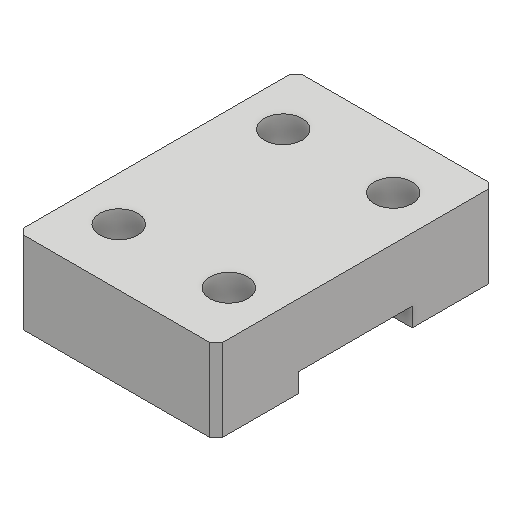
# Autodesk Inventor part: 3DP_ABS_X_Axis_Timing_Belt_Clamp
Saved by Autodesk Inventor 2026.1 (Build 301233000, 233)
## iProperties
Created: 2016-06-18
Part Number: 3DP_ABS_X_Axis_Timing_Belt_Clamp
Material: Ogólny
Document SubType Name: Modeling
Designer: Andrzej
Density: 1 g/cm^3
Appearance: Domyślna
Mass: 1.88495 g
Surface Area: 14.8746 cm^2
Volume: 1.88495 cm^3
Author: Andrzej
Autodesk Inventor part; units mm, degrees
ref_plane "YZ Plane" through (0, 0, 0) normal (1, 0, 0) x (0, 1, 0)
ref_plane "XZ Plane" through (0, 0, 0) normal (0, 1, 0) x (-1, 0, 0)
ref_plane "XY Plane" through (0, 0, 0) normal (0, 0, 1) x (1, 0, 0)
sketch "Szkic1" plane through (0, 0, 0) normal (0, 0, 1) x (1, 0, 0)
  line L0 (-11.2555, 18.1319) -> (4.4445, 18.1319)
  line L1 (4.4445, 18.1319) -> (4.4445, -3.8681)
  line L2 (4.4445, -3.8681) -> (-11.2555, -3.8681)
  line L3 (-11.2555, -3.8681) -> (-11.2555, 18.1319)
  line L4 (-11.2555, 2.6319) -> (4.4445, 2.6319)
  line L5 (-11.2555, 11.6319) -> (4.4445, 11.6319)
  point P0 (0, 0)
  dimension "d0" = 15.7
  dimension "d1" = 22
  dimension "d2" = 9
  dimension "d3" = 6.5
  dimension "d4" = 6.5
  constraints: 12 end point, 4 point on line, 3 perpendicular, 2 parallel, 1 horizontal
  measures "d0" distance of L1.end L2.end
  measures "d1" distance of L2.end L0.start
  measures "d2" distance between parallel lines of L5 L4
  measures "d3" distance between parallel lines of L0 L5
  measures "d4" distance between parallel lines of L2 L4
extrude "Wyciągnięcie proste1" add sketch "Szkic1" along normal blind 1.5 contours L0 L1 L5 L3 | L4 L1 L2 L3
sketch "Szkic2" plane through (0, 0, 1.5) normal (0, 0, 1) x (1, 0, 0)
  line L0 (-11.2555, 18.1319) -> (-11.2555, 11.6319) projected
  line L1 (-11.2555, 18.1319) -> (-11.2555, 11.6319) projected
  line L2 (-11.2555, 11.6319) -> (4.4445, 11.6319) projected
  line L3 (4.4445, 11.6319) -> (4.4445, 18.1319) projected
  line L4 (4.4445, 18.1319) -> (-11.2555, 18.1319) projected
  line L5 (4.4445, -3.8681) -> (4.4445, 2.6319) projected
  line L6 (4.4445, 2.6319) -> (-11.2555, 2.6319) projected
  line L7 (-11.2555, 2.6319) -> (-11.2555, -3.8681) projected
  line L8 (-11.2555, -3.8681) -> (4.4445, -3.8681) projected
  line L9 (4.4445, 18.1319) -> (-11.2555, 18.1319) projected
  line L10 (-11.2555, 18.1319) -> (4.4445, 18.1319)
  line L11 (4.4445, 18.1319) -> (4.4445, -3.8681)
  line L12 (4.4445, -3.8681) -> (-11.2555, -3.8681)
  line L13 (-11.2555, -3.8681) -> (-11.2555, 18.1319)
  point P0 (0, 0)
  constraints: 8 end point, 2 parallel, 1 horizontal, 1 perpendicular
extrude "Wyciągnięcie proste2" add sketch "Szkic2" along normal blind 5
sketch "Szkic3" plane through (0, 0, 6.5) normal (0, 0, 1) x (1, 0, 0)
  line L0 (-11.2555, 11.6319) -> (4.4445, 11.6319) projected
  line L1 (4.4445, 2.6319) -> (-11.2555, 2.6319) projected
  line L2 (-11.2555, 18.1319) -> (-11.2555, -3.8681) projected
  line L3 (-11.2555, -3.8681) -> (4.4445, -3.8681) projected
  line L4 (4.4445, -3.8681) -> (4.4445, 18.1319) projected
  line L5 (4.4445, 18.1319) -> (-11.2555, 18.1319) projected
  point P0 (0, 0)
  point P1 (-7.7555, 13.6319)
  point P2 (0.9445, 13.6319)
  point P3 (-7.7555, 0.6319)
  point P4 (0.9445, 0.6319)
  dimension "d9" = 2
  dimension "d10" = 2
  dimension "d11" = 2
  dimension "d12" = 2
  dimension "d13" = 15.7
  dimension "d14" = 3.5
  dimension "d15" = 3.5
  dimension "d16" = 3.5
  dimension "d17" = 3.5
  measures "d9" distance from line of L0 point (-7.756, 13.632)
  measures "d10" distance from line of L0 point (0.944, 13.632)
  measures "d11" distance from line of L1 point (0.944, 0.632)
  measures "d12" distance from line of L1 point (-7.756, 0.632)
  measures "d13" distance of L4.end L2.start
  measures "d14" distance from line of point (-7.756, 13.632) L2
  measures "d15" distance from line of L4 point (0.944, 13.632)
  measures "d16" distance from line of L4 point (0.944, 0.632)
  measures "d17" distance from line of L2 point (-7.756, 0.632)
hole "Otwór1" at (-7.7555, 13.6319, 6.5) at (0.9445, 13.6319, 6.5) at (-7.7555, 0.6319, 6.5) at (0.9445, 0.6319, 6.5) direction (0, 0, -1) diameter 3 end through all
sketch "Szkic5" plane through (-11.2555, 2.6319, 0) normal (0, 1, 0) x (1, 0, 0)
  line L0 (0, 0) -> (15.7, 0) projected
  line L1 (15.7, 0) -> (15.7, -6.5) projected
  line L2 (0, -6.5) -> (15.7, -6.5) projected
  line L3 (0, 0) -> (0, -6.5) projected
  line L4 (12.8, -0.5) -> (12, -0.5)
  line L5 (12, -0.5) -> (12, -1.5)
  line L6 (10.8, -0.5) -> (10.8, -1.5)
  line L7 (10.8, -0.5) -> (10, -0.5)
  line L8 (10, -0.5) -> (10, -1.5)
  line L9 (8.8, -0.5) -> (8.8, -1.5)
  line L10 (8.8, -0.5) -> (8, -0.5)
  line L11 (8, -0.5) -> (8, -1.5)
  line L12 (6.8, -0.5) -> (6.8, -1.5)
  line L13 (6.8, -0.5) -> (6, -0.5)
  line L14 (6, -0.5) -> (6, -1.5)
  line L15 (4.8, -0.5) -> (4.8, -1.5)
  line L16 (4.8, -0.5) -> (4, -0.5)
  line L17 (4, -0.5) -> (4, -1.5)
  line L18 (2.8, -0.5) -> (2.8, -1.5)
  line L19 (2.8, -0.5) -> (2, -0.5)
  line L20 (2, -0.5) -> (2, -1.5)
  line L21 (0.8, -0.5) -> (0.8, -1.5)
  line L22 (0.8, -0.5) -> (0, -0.5)
  line L23 (12.8, -0.5) -> (12.8, -1.5)
  line L24 (14, -1.5) -> (14, -0.5)
  line L25 (14, -0.5) -> (14.8, -0.5)
  line L26 (14.8, -0.5) -> (14.8, -1.5)
  line L27 (0, -1.5) -> (0.8, -1.5)
  line L28 (2, -1.5) -> (2.8, -1.5)
  line L29 (4, -1.5) -> (4.8, -1.5)
  line L30 (6, -1.5) -> (6.8, -1.5)
  line L31 (8, -1.5) -> (8.8, -1.5)
  line L32 (10, -1.5) -> (10.8, -1.5)
  line L33 (12, -1.5) -> (12.8, -1.5)
  line L34 (14, -1.5) -> (14.8, -1.5)
  line L35 (0, -1.5) -> (0, -0.5)
  line L36 (0, 0) -> (0, -6.5) projected
  point P0 (11.2555, 0)
  dimension "d27" = 0.8
  dimension "d28" = 1.2
  dimension "d41" = 1
  dimension "d42" = 0.5
  dimension "d43" = 0.5
  dimension "d44" = 0.5
  dimension "d45" = 0.5
  dimension "d46" = 0.5
  dimension "d47" = 0.5
  dimension "d48" = 0.5
  dimension "d49" = 0.5
  dimension "d50" = 1
  constraints: 64 end point, 16 perpendicular, 9 horizontal, 1 collinear, 1 point on line, 1 vertical
  measures "d27" distance of L24.end L25.end
  measures "d28" distance between parallel lines of L24 L23
  measures "d41" distance of L25.end L26.end
  measures "d42" distance between parallel lines of L0 L25
  measures "d43" distance between parallel lines of L0 L4
  measures "d44" distance between parallel lines of L0 L7
  measures "d45" distance between parallel lines of L0 L10
  measures "d46" distance between parallel lines of L0 L13
  measures "d47" distance between parallel lines of L0 L16
  measures "d48" distance between parallel lines of L0 L19
  measures "d49" distance between parallel lines of L0 L22
  measures "d50" distance between parallel lines of L22 L27
extrude "Wyciągnięcie proste3" add sketch "Szkic5" along normal blind 9 contours L22 L21 L27 L3 | L23 L33 L5 L4 | L6 L32 L8 L7 | L9 L31 L11 L10 | L12 L30 L14 L13 | L15 L29 L17 L16 | L18 L28 L20 L19 | L24 L25 L26 L34
fillet "Zaokrąglenie1" radius 0.2 16 edges at (-9.2555, 7.1319, 0.5) (-8.4555, 7.1319, 0.5) (-7.2555, 7.1319, 0.5) (-6.4555, 7.1319, 0.5) (-5.2555, 7.1319, 0.5) (-4.4555, 7.1319, 0.5) (-3.2555, 7.1319, 0.5) (-2.4555, 7.1319, 0.5) (-1.2555, 7.1319, 0.5) (-0.4555, 7.1319, 0.5) (0.7445, 7.1319, 0.5) (1.5445, 7.1319, 0.5) (2.7445, 7.1319, 0.5) (3.5445, 7.1319, 0.5) (-10.4555, 7.1319, 0.5) (-11.2555, 7.1319, 0.5)
chamfer "Faza1" distance 0.5 angle 45 4 edges at (-11.2555, -3.8681, 3.25) (4.4445, -3.8681, 3.25) (-11.2555, 18.1319, 3.25) (4.4445, 18.1319, 3.25)
equation "\"d10\" = d9"
equation "\"d11\" = d9"
equation "\"d12\" = d9"
equation "\"d15\" = d14"
equation "\"d16\" = d14"
equation "\"d17\" = d14"
equation "\"d43\" = d42"
equation "\"d44\" = d42"
equation "\"d45\" = d42"
equation "\"d46\" = d42"
equation "\"d47\" = d42"
equation "\"d48\" = d42"
equation "\"d49\" = d42"
